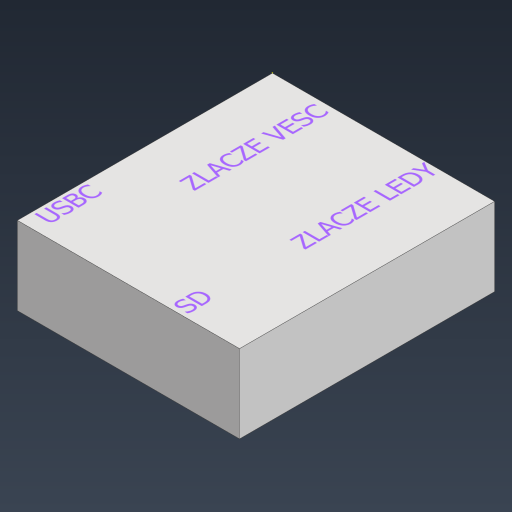
# Autodesk Inventor part: MKS_express
Saved by Autodesk Inventor 2023 (Build 270158000, 158)
## iProperties
Created: 2025-12-27
Part Number: MKS_express
Material: Generic
Document SubType Name: Modeling
Designer: szymo
Density: 1 g/cm^3
Appearance: Default
Author: szymo
Autodesk Inventor part; units mm, degrees
ref_plane "YZ Plane" through (0, 0, 0) normal (1, 0, 0) x (0, 1, 0)
ref_plane "XZ Plane" through (0, 0, 0) normal (0, 1, 0) x (-1, 0, 0)
ref_plane "XY Plane" through (0, 0, 0) normal (0, 0, 1) x (1, 0, 0)
sketch "Sketch1" plane through (0, 0, 0) normal (0, 1, 0) x (-1, 0, 0)
  line L0 (0, 0) -> (-27, 0)
  line L1 (-27, 0) -> (-27, 31)
  line L2 (-27, 31) -> (0, 31)
  line L3 (0, 31) -> (0, 0)
  dimension "d0" = 27
  dimension "d1" = 31
  constraints: 8 end point, 2 parallel, 1 horizontal, 1 perpendicular
  measures "d0" distance of L1.end L2.end
  measures "d1" distance of L0.end L1.end
extrude "Extrusion1" add sketch "Sketch1" along normal blind 9.5
sketch "Sketch2" plane through (0, 9.5, 0) normal (0, 1, 0) x (1, 0, 0)
  line L0 (0.3486, -29.4936) -> (0.3486, -19.4233) construction
  line L1 (0.3486, -19.4233) -> (3.5152, -19.4233) construction
  line L2 (3.5152, -19.4233) -> (3.5152, -29.4936) construction
  line L3 (3.5152, -29.4936) -> (0.3486, -29.4936) construction
  line L4 (5.6321, -17.1808) -> (5.6321, 7.9887) construction
  line L5 (5.6321, 7.9887) -> (8.7887, 7.9887) construction
  line L6 (8.7887, 7.9887) -> (8.7887, -17.1808) construction
  line L7 (8.7887, -17.1808) -> (5.6321, -17.1808) construction
  line L8 (18.5381, -16.6448) -> (18.5381, 8.5642) construction
  line L9 (18.5381, 8.5642) -> (21.6948, 8.5642) construction
  line L10 (21.6948, 8.5642) -> (21.6948, -16.6448) construction
  line L11 (21.6948, -16.6448) -> (18.5381, -16.6448) construction
  line L12 (18.1944, -30.5524) -> (18.1944, -25.3753) construction
  line L13 (18.1944, -25.3753) -> (21.3511, -25.3753) construction
  line L14 (21.3511, -25.3753) -> (21.3511, -30.5524) construction
  line L15 (21.3511, -30.5524) -> (18.1944, -30.5524) construction
  point P0 (0, 0)
  constraints: 8 other
body "Solid1"
